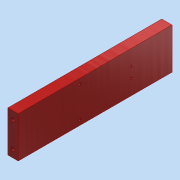
# Autodesk Inventor part: side_panel
Saved by Autodesk Inventor 2022 (Build 260153000, 153)
## iProperties
Created: 2020-09-20
Part Number: side_panel
Material: Generic
Document SubType Name: Modeling
Designer: nnico
Density: 1 g/cm^3
Appearance: Red
Author: nnico
Autodesk Inventor part; units mm, degrees
ref_plane "YZ Plane" through (0, 0, 0) normal (1, 0, 0) x (0, 1, 0)
ref_plane "XZ Plane" through (0, 0, 0) normal (0, 1, 0) x (-1, 0, 0)
ref_plane "XY Plane" through (0, 0, 0) normal (0, 0, 1) x (1, 0, 0)
sketch "Sketch1" plane through (0, 0, 0) normal (0, 1, 0) x (-1, 0, 0)
  line L0 (10, 40) -> (-10, 40)
  line L1 (-10, 40) -> (-10, -40)
  line L2 (-10, -40) -> (10, -40)
  line L3 (10, -40) -> (10, 40)
  line L4 (10, 0) -> (-10, 0) construction
  line L5 (0, 40) -> (0, -40) construction
  point P0 (0, 0)
  point P1 (0, 0)
  dimension "d0" = 20
  dimension "d1" = 80
  constraints: 12 end point, 5 midpoint, 2 parallel, 1 coincident, 1 horizontal, 1 perpendicular
  measures "d0" distance of L0.start L0.end
  measures "d1" distance of L2.end L0.start
extrude "Extrusion1" add sketch "Sketch1" along normal blind 300
sketch "Sketch2" plane through (0, 300, 0) normal (0, 1, 0) x (1, 0, 0)
  circle A0 centre (0, 25) radius 3.5
  circle A1 centre (0, -25) radius 3.5
  line L0 (0, -25) -> (0, 25) construction
  line L1 (10, 40) -> (-10, 40) construction
  line L2 (0, 40) -> (0, -40) construction
  line L3 (-10, -40) -> (10, -40) construction
  point P0 (0, 0)
  dimension "d4" = 7
  dimension "d5" = 7
  dimension "d6" = 50
  dimension "d7" = 15
  constraints: 4 end point, 2 centre point, 2 midpoint, 1 point on line, 1 vertical
  measures "d4" diameter of A0
  measures "d5" diameter of A1
  measures "d6" distance of L0.start L0.end
  measures "d7" distance from line of L1 L0.end
extrude "Extrusion2" cut sketch "Sketch2" against normal blind 12
sketch "Sketch3" plane through (0, 0, 0) normal (0, -1, 0) x (1, 0, 0)
  circle A0 centre (0, 25) radius 3.5 projected
  circle A1 centre (0, -25) radius 3.5 projected
  point P0 (0, 0)
extrude "Extrusion3" cut sketch "Sketch3" against normal blind 12
sketch "Sketch4" plane through (-10, 0, -40) normal (-1, 0, 0) x (0, 0, 1)
  circle A0 centre (10, 120) radius 2.25
  circle A1 centre (70, 120) radius 2.25
  line L0 (10, 120) -> (70, 120) construction
  line L1 (0, 0) -> (0, 300) construction
  line L2 (0, 0) -> (80, 0) construction
  point P0 (40, 0)
  dimension "d12" = 4.5
  dimension "d13" = 4.5
  dimension "d14" = 60
  dimension "d15" = 10
  dimension "d16" = 120
  constraints: 2 centre point, 2 end point, 1 horizontal
  measures "d12" diameter of A0
  measures "d13" diameter of A1
  measures "d14" distance of L0.start L0.end
  measures "d15" distance from line of L1 L0.start
  measures "d16" distance from line of L2 L0.end
extrude "Extrusion4" cut sketch "Sketch4" against normal up to next
sketch "Sketch5" plane through (-10, 0, -40) normal (-1, 0, 0) x (0, 0, 1)
  circle A0 centre (30, 220) radius 1.75
  circle A1 centre (50, 220) radius 1.75
  line L0 (30, 220) -> (50, 220) construction
  line L1 (0, 0) -> (0, 300) construction
  line L2 (0, 300) -> (80, 300) construction
  point P0 (40, 0)
  dimension "d19" = 3.5
  dimension "d20" = 3.5
  dimension "d21" = 20
  dimension "d22" = 30
  dimension "d23" = 80
  constraints: 2 centre point, 2 end point, 1 horizontal
  measures "d19" diameter of A0
  measures "d20" diameter of A1
  measures "d21" distance of L0.start L0.end
  measures "d22" distance from line of L1 L0.start
  measures "d23" distance from line of L2 L0.start
extrude "Extrusion5" cut sketch "Sketch5" against normal up to next
body "Solid1"
